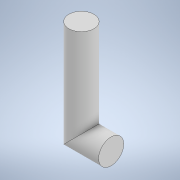
# Autodesk Inventor part: Placeholder_For_Bevel_Gear
Saved by Autodesk Inventor 2022 (Build 260153000, 153)
## iProperties
Created: 2022-04-04
Part Number: Placeholder_For_Bevel_Gear
Material: Generic
Document SubType Name: Modeling
Designer: Mlees
Density: 1 g/cm^3
Appearance: Default
Author: Mlees
Autodesk Inventor part; units mm, degrees
ref_plane "YZ Plane" through (0, 0, 0) normal (1, 0, 0) x (0, 1, 0)
ref_plane "XZ Plane" through (0, 0, 0) normal (0, 1, 0) x (-1, 0, 0)
ref_plane "XY Plane" through (0, 0, 0) normal (0, 0, 1) x (1, 0, 0)
sketch "Sketch1" plane through (0, 0, 0) normal (1, 0, 0) x (0, 1, 0)
  circle A0 centre (0, 0) radius 2.5
  dimension "d0" = 5
  constraints: 1 centre point, 1 coincident
  measures "d0" diameter of A0
sketch "Sketch2" plane through (0, 0, 0) normal (0, 0, 1) x (1, 0, 0)
  line L0 (0, 0) -> (-5.927, 0)
  line L1 (-5.927, 19.4159) -> (-5.927, 0)
  dimension "d1" = 5.927
  dimension "d5" = 19.4159
  constraints: 4 end point, 1 horizontal, 1 vertical
  measures "d1" distance of L0.start L0.end
  measures "d5" distance of L1.start L0.end
sweep "Sweep1" add profiles "Sketch1" path "Sketch2"
body "Solid1"
